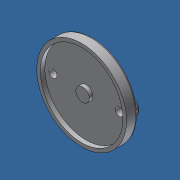
# Autodesk Inventor part: PAD 100mm GRAY PLASTIC WITH ATTACHMENT BORES
Saved by Autodesk Inventor 2016 (Build 200138000, 138)
## iProperties
Created: 2007-03-28
Part Number: PAD 100mm GRAY PLASTIC WITH ATTACHMENT BORES
Document SubType Name: Modeling
Designer: Andy Moles
Material: ABS Plastic
Density: 1.06 g/cm^3
Appearance: Light Gray
Author: Andy Moles
Autodesk Inventor part; units mm, degrees
ref_plane "YZ Plane" through (0, 0, 0) normal (1, 0, 0) x (0, 1, 0)
ref_plane "XZ Plane" through (0, 0, 0) normal (0, 1, 0) x (-1, 0, 0)
ref_plane "XY Plane" through (0, 0, 0) normal (0, 0, 1) x (1, 0, 0)
sketch "Sketch1" plane through (0, 0, 0) normal (0, 0, 1) x (1, 0, 0)
  line L0 (0, 0) -> (50, 0)
  line L1 (50, 0) -> (50, 10.3348)
  line L2 (0, 0) -> (0, 19) construction
  arc A0 (0, 8) -> (6.6332, 19) centre (0, 15.5) ccw
  line L3 (6.6332, 19) -> (11.8173, 19)
  line L4 (48.3623, 12.3017) -> (12.1797, 18.9669)
  arc A1 (12.1797, 18.9669) -> (11.8173, 19) centre (11.8173, 17) ccw
  arc A2 (50, 10.3348) -> (48.3623, 12.3017) centre (48, 10.3348) ccw
  line L5 (0, 0) -> (0, 8)
  point P0 (50, 12)
  point P1 (12, 19)
  dimension "d0" = 50
  dimension "d1" = 12
  dimension "d2" = 19
  dimension "d3" = 15
  dimension "d4" = 3.5
  dimension "d5" = 12
  dimension "d6" = 2
  dimension "d14" = 19
  constraints: 12 end point, 6 point on circle, 6 point on line, 4 tangent, 3 centre point, 2 perpendicular, 1 collinear, 1 equal radius, 1 horizontal, 1 parallel
  measures "d0" distance of L0.start L0.end
  measures "d1" distance of L0.end point (50, 12)
  measures "d2" distance of L0.start L2.end
  measures "d3" diameter of A0
  measures "d4" distance of A0.centre L2.end
  measures "d5" horizontal distance of point (12, 19) L0.start
  measures "d6" radius of A1
  measures "d14" distance between parallel lines of L3 L0
revolve "Revolution1" add sketch "Sketch1" angle 360 about axis through (0, 0, 0) along (0, 1, 0)
sketch "Sketch2" plane through (0, 0, 0) normal (0, -1, 0) x (1, 0, 0)
  circle A0 centre (0, 0) radius 50 projected
  circle A1 centre (0, 0) radius 7.5
  dimension "d8" = 15
  constraints: 1 centre point, 1 coincident
  measures "d8" diameter of A1
extrude "Extrusion1" cut sketch "Sketch2" against normal blind 1 contours A1
sketch "Sketch3" plane through (0, 0, 0) normal (0, -1, 0) x (1, 0, 0)
  circle A0 centre (0, 0) radius 7.5 projected
  circle A1 centre (0, 0) radius 50 projected
  circle A2 centre (0, 0) radius 46
  dimension "d11" = 4
  constraints: 1 centre point, 1 coincident
  measures "d11" radial gap between concentric circles of A1 A2
extrude "Extrusion2" cut sketch "Sketch3" against normal blind 5 contours A2
sketch "Sketch4" plane through (0, 5, 0) normal (0, -1, 0) x (1, 0, 0)
  circle A0 centre (0, 0) radius 7.5 projected
  arc A1 (-37, 10) -> (-37, -10) centre (-37, 0) ccw
  arc A2 (37, -10) -> (37, 10) centre (37, 0) ccw
  line L0 (12, 10) -> (12, -10)
  line L1 (-12, 10) -> (-12, -10)
  line L2 (-37, 10) -> (-12, 10)
  line L3 (-37, -10) -> (-12, -10)
  line L4 (12, 10) -> (37, 10)
  line L5 (12, -10) -> (37, -10)
  point P0 (-12, 0)
  point P1 (12, 0)
  dimension "d15" = 20
  dimension "d16" = 20
  dimension "d17" = 74
  dimension "d18" = 37
  dimension "d19" = 20
  dimension "d20" = 20
  dimension "d21" = 25
  dimension "d22" = 25
  constraints: 12 end point, 4 horizontal alignment, 4 point on circle, 3 parallel, 2 centre point, 2 midpoint, 1 perpendicular, 1 tangent, 1 vertical
  measures "d15" diameter of A1
  measures "d16" diameter of A2
  measures "d17" distance of A2.centre A1.centre
  measures "d18" distance of A0.centre A1.centre
  measures "d19" distance of L1.start L1.end
  measures "d20" distance of L0.start L0.end
  measures "d21" distance from line of L1 A1.centre
  measures "d22" distance from line of L0 A2.centre
extrude "Extrusion3" add sketch "Sketch4" against normal blind 13 contours L2 L1 L3 A1 | L5 L0 L4 A2
fillet "Fillet1" radius 2 6 edges at (-25.6371, 18, 10) (-47, 18, 0) (-25.6371, 18, -10) (25.6371, 18, 10) (47, 18, 0) (25.6371, 18, -10)
sketch "Sketch5" plane through (0, 5, 0) normal (0, -1, 0) x (1, 0, 0)
  arc A0 (-37, 10) -> (-37, -10) centre (-37, 0) ccw projected
  circle A1 centre (-37, 0) radius 4.5
  circle A2 centre (37, 0) radius 4.5
  dimension "d26" = 9
  dimension "d27" = 9
  constraints: 2 centre point, 2 coincident
  measures "d26" diameter of A1
  measures "d27" diameter of A2
extrude "Extrusion4" cut sketch "Sketch5" against normal through all
equation "\"d18\" = 0.5 * d17"
equation "\"d22\" = d21"
equation "\"d27\" = d26"
body "Solid1"
